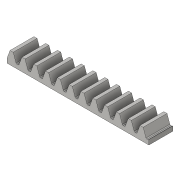
# Autodesk Inventor part: Rack
Saved by Autodesk Inventor 2016 (Build 200138000, 138)
## iProperties
Created: 2016-04-02
Part Number: Rack
Material: Generic
Document SubType Name: Modeling
Designer: amycroft3
Density: 1 g/cm^3
Appearance: Default
Author: amycroft3
Autodesk Inventor part; units mm, degrees
ref_plane "YZ Plane" through (0, 0, 0) normal (1, 0, 0) x (0, 1, 0)
ref_plane "XZ Plane" through (0, 0, 0) normal (0, 1, 0) x (-1, 0, 0)
ref_plane "XY Plane" through (0, 0, 0) normal (0, 0, 1) x (1, 0, 0)
sketch "Sketch1" plane through (0, 0, 0) normal (0, 0, 1) x (1, 0, 0)
  line L0 (27.361, 9.329) -> (25.8429, 13.5)
  line L1 (25.8429, 13.5) -> (24.1571, 13.5)
  line L2 (24.1571, 13.5) -> (22.639, 9.329)
  arc A0 (22.1692, 9) -> (22.639, 9.329) centre (22.1692, 9.5) ccw
  line L3 (22.1692, 9) -> (0, 9)
  line L4 (0, 9) -> (0, 0)
  line L5 (0, 0) -> (175.6637, 0)
  line L6 (175.6637, 0) -> (175.6637, 9)
  line L7 (175.6637, 9) -> (153.4945, 9)
  arc A1 (153.0247, 9.329) -> (153.4945, 9) centre (153.4945, 9.5) ccw
  line L8 (153.0247, 9.329) -> (151.5066, 13.5)
  line L9 (151.5066, 13.5) -> (149.8209, 13.5)
  line L10 (149.8209, 13.5) -> (148.3027, 9.329)
  arc A2 (147.8329, 9) -> (148.3027, 9.329) centre (147.8329, 9.5) ccw
  line L11 (147.8329, 9) -> (147.2113, 9)
  arc A3 (146.7415, 9.329) -> (147.2113, 9) centre (147.2113, 9.5) ccw
  line L12 (146.7415, 9.329) -> (145.2234, 13.5)
  line L13 (145.2234, 13.5) -> (143.5377, 13.5)
  line L14 (143.5377, 13.5) -> (142.0195, 9.329)
  arc A4 (141.5497, 9) -> (142.0195, 9.329) centre (141.5497, 9.5) ccw
  line L15 (141.5497, 9) -> (140.9282, 9)
  arc A5 (140.4583, 9.329) -> (140.9282, 9) centre (140.9282, 9.5) ccw
  line L16 (140.4583, 9.329) -> (138.9402, 13.5)
  line L17 (138.9402, 13.5) -> (137.2545, 13.5)
  line L18 (137.2545, 13.5) -> (135.7364, 9.329)
  arc A6 (135.2665, 9) -> (135.7364, 9.329) centre (135.2665, 9.5) ccw
  line L19 (135.2665, 9) -> (134.645, 9)
  arc A7 (134.1751, 9.329) -> (134.645, 9) centre (134.645, 9.5) ccw
  line L20 (134.1751, 9.329) -> (132.657, 13.5)
  line L21 (132.657, 13.5) -> (130.9713, 13.5)
  line L22 (130.9713, 13.5) -> (129.4532, 9.329)
  arc A8 (128.9833, 9) -> (129.4532, 9.329) centre (128.9833, 9.5) ccw
  line L23 (128.9833, 9) -> (128.3618, 9)
  arc A9 (127.8919, 9.329) -> (128.3618, 9) centre (128.3618, 9.5) ccw
  line L24 (127.8919, 9.329) -> (126.3738, 13.5)
  line L25 (126.3738, 13.5) -> (124.6881, 13.5)
  line L26 (124.6881, 13.5) -> (123.17, 9.329)
  arc A10 (122.7001, 9) -> (123.17, 9.329) centre (122.7001, 9.5) ccw
  line L27 (122.7001, 9) -> (122.0786, 9)
  arc A11 (121.6088, 9.329) -> (122.0786, 9) centre (122.0786, 9.5) ccw
  line L28 (121.6088, 9.329) -> (120.0906, 13.5)
  line L29 (120.0906, 13.5) -> (118.4049, 13.5)
  line L30 (118.4049, 13.5) -> (116.8868, 9.329)
  arc A12 (116.417, 9) -> (116.8868, 9.329) centre (116.417, 9.5) ccw
  line L31 (116.417, 9) -> (115.7954, 9)
  arc A13 (115.3256, 9.329) -> (115.7954, 9) centre (115.7954, 9.5) ccw
  line L32 (115.3256, 9.329) -> (113.8075, 13.5)
  line L33 (113.8075, 13.5) -> (112.1217, 13.5)
  line L34 (112.1217, 13.5) -> (110.6036, 9.329)
  arc A14 (110.1338, 9) -> (110.6036, 9.329) centre (110.1338, 9.5) ccw
  line L35 (110.1338, 9) -> (109.5122, 9)
  arc A15 (109.0424, 9.329) -> (109.5122, 9) centre (109.5122, 9.5) ccw
  line L36 (109.0424, 9.329) -> (107.5243, 13.5)
  line L37 (107.5243, 13.5) -> (105.8386, 13.5)
  line L38 (105.8386, 13.5) -> (104.3204, 9.329)
  arc A16 (103.8506, 9) -> (104.3204, 9.329) centre (103.8506, 9.5) ccw
  line L39 (103.8506, 9) -> (103.229, 9)
  arc A17 (102.7592, 9.329) -> (103.229, 9) centre (103.229, 9.5) ccw
  line L40 (102.7592, 9.329) -> (101.2411, 13.5)
  line L41 (101.2411, 13.5) -> (99.5554, 13.5)
  line L42 (99.5554, 13.5) -> (98.0372, 9.329)
  arc A18 (97.5674, 9) -> (98.0372, 9.329) centre (97.5674, 9.5) ccw
  line L43 (97.5674, 9) -> (96.9459, 9)
  arc A19 (96.476, 9.329) -> (96.9459, 9) centre (96.9459, 9.5) ccw
  line L44 (96.476, 9.329) -> (94.9579, 13.5)
  line L45 (94.9579, 13.5) -> (93.2722, 13.5)
  line L46 (93.2722, 13.5) -> (91.7541, 9.329)
  arc A20 (91.2842, 9) -> (91.7541, 9.329) centre (91.2842, 9.5) ccw
  line L47 (91.2842, 9) -> (90.6627, 9)
  arc A21 (90.1928, 9.329) -> (90.6627, 9) centre (90.6627, 9.5) ccw
  line L48 (90.1928, 9.329) -> (88.6747, 13.5)
  line L49 (88.6747, 13.5) -> (86.989, 13.5)
  line L50 (86.989, 13.5) -> (85.4709, 9.329)
  arc A22 (85.001, 9) -> (85.4709, 9.329) centre (85.001, 9.5) ccw
  line L51 (85.001, 9) -> (84.3795, 9)
  arc A23 (83.9096, 9.329) -> (84.3795, 9) centre (84.3795, 9.5) ccw
  line L52 (83.9096, 9.329) -> (82.3915, 13.5)
  line L53 (82.3915, 13.5) -> (80.7058, 13.5)
  line L54 (80.7058, 13.5) -> (79.1877, 9.329)
  arc A24 (78.7178, 9) -> (79.1877, 9.329) centre (78.7178, 9.5) ccw
  line L55 (78.7178, 9) -> (78.0963, 9)
  arc A25 (77.6265, 9.329) -> (78.0963, 9) centre (78.0963, 9.5) ccw
  line L56 (77.6265, 9.329) -> (76.1083, 13.5)
  line L57 (76.1083, 13.5) -> (74.4226, 13.5)
  line L58 (74.4226, 13.5) -> (72.9045, 9.329)
  arc A26 (72.4347, 9) -> (72.9045, 9.329) centre (72.4347, 9.5) ccw
  line L59 (72.4347, 9) -> (71.8131, 9)
  arc A27 (71.3433, 9.329) -> (71.8131, 9) centre (71.8131, 9.5) ccw
  line L60 (71.3433, 9.329) -> (69.8252, 13.5)
  line L61 (69.8252, 13.5) -> (68.1394, 13.5)
  line L62 (68.1394, 13.5) -> (66.6213, 9.329)
  arc A28 (66.1515, 9) -> (66.6213, 9.329) centre (66.1515, 9.5) ccw
  line L63 (66.1515, 9) -> (65.5299, 9)
  arc A29 (65.0601, 9.329) -> (65.5299, 9) centre (65.5299, 9.5) ccw
  line L64 (65.0601, 9.329) -> (63.542, 13.5)
  line L65 (63.542, 13.5) -> (61.8563, 13.5)
  line L66 (61.8563, 13.5) -> (60.3381, 9.329)
  arc A30 (59.8683, 9) -> (60.3381, 9.329) centre (59.8683, 9.5) ccw
  line L67 (59.8683, 9) -> (59.2468, 9)
  arc A31 (58.7769, 9.329) -> (59.2468, 9) centre (59.2468, 9.5) ccw
  line L68 (58.7769, 9.329) -> (57.2588, 13.5)
  line L69 (57.2588, 13.5) -> (55.5731, 13.5)
  line L70 (55.5731, 13.5) -> (54.0549, 9.329)
  arc A32 (53.5851, 9) -> (54.0549, 9.329) centre (53.5851, 9.5) ccw
  line L71 (53.5851, 9) -> (52.9636, 9)
  arc A33 (52.4937, 9.329) -> (52.9636, 9) centre (52.9636, 9.5) ccw
  line L72 (52.4937, 9.329) -> (50.9756, 13.5)
  line L73 (50.9756, 13.5) -> (49.2899, 13.5)
  line L74 (49.2899, 13.5) -> (47.7718, 9.329)
  arc A34 (47.3019, 9) -> (47.7718, 9.329) centre (47.3019, 9.5) ccw
  line L75 (47.3019, 9) -> (46.6804, 9)
  arc A35 (46.2105, 9.329) -> (46.6804, 9) centre (46.6804, 9.5) ccw
  line L76 (46.2105, 9.329) -> (44.6924, 13.5)
  line L77 (44.6924, 13.5) -> (43.0067, 13.5)
  line L78 (43.0067, 13.5) -> (41.4886, 9.329)
  arc A36 (41.0187, 9) -> (41.4886, 9.329) centre (41.0187, 9.5) ccw
  line L79 (41.0187, 9) -> (40.3972, 9)
  arc A37 (39.9273, 9.329) -> (40.3972, 9) centre (40.3972, 9.5) ccw
  line L80 (39.9273, 9.329) -> (38.4092, 13.5)
  line L81 (38.4092, 13.5) -> (36.7235, 13.5)
  line L82 (36.7235, 13.5) -> (35.2054, 9.329)
  arc A38 (34.7355, 9) -> (35.2054, 9.329) centre (34.7355, 9.5) ccw
  line L83 (34.7355, 9) -> (34.114, 9)
  arc A39 (33.6442, 9.329) -> (34.114, 9) centre (34.114, 9.5) ccw
  line L84 (33.6442, 9.329) -> (32.126, 13.5)
  line L85 (32.126, 13.5) -> (30.4403, 13.5)
  line L86 (30.4403, 13.5) -> (28.9222, 9.329)
  arc A40 (28.4524, 9) -> (28.9222, 9.329) centre (28.4524, 9.5) ccw
  line L87 (28.4524, 9) -> (27.8308, 9)
  arc A41 (27.361, 9.329) -> (27.8308, 9) centre (27.8308, 9.5) ccw
  point P0 (87.8319, 5)
  constraints: 176 end point, 84 point on circle, 42 centre point
extrude "Extrusion1" add sketch "Sketch1" along normal blind 12.7
sketch "Sketch2" plane through (0, 0, 12.7) normal (0, 0, 1) x (1, 0, 0)
  line L0 (0, 9) -> (22.1692, 9) projected
  line L1 (175.6637, 9) -> (153.4945, 9) projected
  line L2 (0, 9) -> (175.6637, 9)
  point P0 (0, 0)
  constraints: 2 end point, 1 horizontal
sketch "Sketch3" plane through (0, 0, 12.7) normal (0, 0, 1) x (1, 0, 0)
  line L0 (22.639, 9.329) -> (24.1571, 13.5) projected
  line L1 (175.6637, 0) -> (0, 0) projected
  line L2 (22.639, 9.329) -> (0, 9.329)
  line L3 (0, 9.329) -> (0, 0)
  line L4 (0, 0) -> (22.639, 0)
  line L5 (22.639, 0) -> (22.639, 9.329)
  line L6 (22.639, 0) -> (98.839, 0)
  line L7 (98.0372, 13.6919) -> (175.6637, 13.6919)
  line L8 (175.6637, 13.6919) -> (175.6637, 0)
  line L9 (175.6637, 0) -> (98.0372, 0)
  line L10 (98.0372, 0) -> (98.0372, 13.6919)
  line L11 (22.639, 0) -> (98.0372, 0)
  line L12 (98.0372, 0) -> (98.0372, 6.846)
  line L13 (98.0372, 6.846) -> (22.639, 6.846)
  line L14 (22.639, 6.846) -> (22.639, 0)
  dimension "d3" = 13.6919
  dimension "d4" = 77.6265
  dimension "d5" = 74.7953
  constraints: 26 end point, 6 parallel, 4 horizontal, 3 perpendicular, 1 midpoint
  measures "d3" distance between parallel lines of L7 L1
  measures "d4" distance between parallel lines of L8 L10
  measures "d5" distance from line of L6.end L0
extrude "Extrusion2" cut sketch "Sketch3" against normal blind 25.4
body "Solid1"
